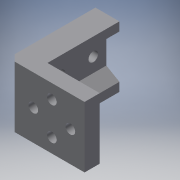
# Autodesk Inventor part: Test Mount
Saved by Autodesk Inventor 2017 (Build 210142000, 142)
## iProperties
Created: 2017-09-01
Part Number: Test Mount
Material: Generic
Document SubType Name: Modeling
Designer: Thein Lin Aung
Density: 1 g/cm^3
Appearance: Default
Author: Thein Lin Aung
Autodesk Inventor part; units mm, degrees
ref_plane "YZ Plane" through (0, 0, 0) normal (1, 0, 0) x (0, 1, 0)
ref_plane "XZ Plane" through (0, 0, 0) normal (0, 1, 0) x (-1, 0, 0)
ref_plane "XY Plane" through (0, 0, 0) normal (0, 0, 1) x (1, 0, 0)
sketch "Sketch1" plane through (0, 0, 0) normal (0, 0, 1) x (1, 0, 0)
  line L0 (35, 0) -> (0, 0)
  line L1 (0, 0) -> (0, 40)
  line L2 (0, 40) -> (5, 40)
  line L3 (5, 40) -> (5, 7)
  line L4 (5, 7) -> (35, 7)
  line L5 (35, 7) -> (35, 0)
  line L6 (-7, 0) -> (42, 0) projected
  line L7 (0, -8) -> (0, 48) projected
  dimension "d0" = 7
  dimension "d1" = 5
  dimension "d2" = 40
  dimension "d3" = 30
  constraints: 13 end point, 5 perpendicular, 1 horizontal
  measures "d0" distance of L4.end L0.start
  measures "d1" distance of L1.end L2.end
  measures "d2" distance of L0.end L1.end
  measures "d3" distance of L3.end L4.end
extrude "Extrusion1" add sketch "Sketch1" along normal mid plane 28
sketch "Sketch2" plane through (5, 7, 14) normal (0, 1, 0) x (1, 0, 0)
  circle A0 centre (15, 21.5) radius 2.2 projected
  circle A1 centre (23.5, 14) radius 2.2 projected
  circle A2 centre (15, 6.5) radius 2.2 projected
  circle A3 centre (6.5, 14) radius 2.2 projected
  point P0 (-5, 14)
extrude "Extrusion2" cut sketch "Sketch2" against normal through all
sketch "Sketch3" plane through (5, 7, 14) normal (0, 1, 0) x (1, 0, 0)
  circle A0 centre (15, 6.5) radius 2.2 projected
  circle A1 centre (15, 21.5) radius 2.2 projected
  circle A2 centre (23.5, 14) radius 2.2 projected
  circle A3 centre (6.5, 14) radius 2.2 projected
  line L0 (0, 28) -> (0, 0) projected
  line L1 (30, 0) -> (0, 0) projected
  line L2 (30, 28) -> (30, 0) projected
  line L3 (0, 28) -> (30, 28) projected
  circle A4 centre (6.5, 14) radius 3.6
  circle A5 centre (15, 21.5) radius 3.6
  circle A6 centre (23.5, 14) radius 2.2 projected
  circle A7 centre (23.5, 14) radius 3.6
  circle A8 centre (15, 6.5) radius 3.6
  point P0 (-5, 14)
  dimension "d8" = 7.2
  constraints: 4 centre point, 4 coincident, 3 equal radius
  measures "d8" diameter of A4
extrude "Extrusion3" cut sketch "Sketch3" against normal blind 4 contours A4 | A5 | A7 | A8
chamfer "Chamfer1" distance 3 angle 45 1 edges at (5, 7, 0)
sketch "Sketch4" plane through (5, 40, 14) normal (1, 0, 0) x (0, 0, -1)
  line L0 (28, 0) -> (0, 0) projected
  line L1 (14, 0) -> (14, -21)
  circle A0 centre (14, -21) radius 2.2
  circle A1 centre (14, -6) radius 2.2
  point P0 (14, -40)
  dimension "d14" = 4.4
  dimension "d15" = 15
  dimension "d16" = 6
  constraints: 2 centre point, 2 end point, 1 coincident, 1 equal radius, 1 midpoint, 1 point on line, 1 vertical
  measures "d14" diameter of A0
  measures "d15" distance of A1.centre L1.end
  measures "d16" distance from line of L0 A1.centre
extrude "Extrusion4" cut sketch "Sketch4" against normal through all
chamfer "Chamfer2" distance 3 angle 45 1 edges at (0, 0, 0)
sketch "Sketch5" plane through (0, 40, 14) normal (0, 1, 0) x (1, 0, 0)
  line L0 (5, 28) -> (5, 0) projected
  line L1 (5, 28) -> (11, 28)
  line L2 (35, 28) -> (3, 28) projected
  line L3 (11, 24) -> (5, 20.5359)
  line L4 (11, 28) -> (11, 24)
  point P0 (0, 14)
  dimension "d22" = 60
  dimension "d23" = 6
  dimension "d24" = 4
  constraints: 6 end point, 2 point on line, 1 perpendicular
  measures "d22" angle of L0 L3
  measures "d23" distance of L0.start L1.end
  measures "d24" distance of L1.end L3.start
extrude "Extrusion5" add sketch "Sketch5" against normal up to surface (33 mm away)
mirror "Mirror1" about plane through (0, 0, 0) normal (0, 0, 1) of "Extrusion5"
sketch "Sketch6" plane through (0, 40, -14) normal (-1, 0, 0) x (0, 0, 1)
  line L0 (0, 0) -> (28, 0) projected
  line L1 (8, 0) -> (20, 0)
  line L2 (20, 0) -> (20, -26)
  line L3 (20, -26) -> (8, -26)
  line L4 (8, -26) -> (8, 0)
  circle A0 centre (14, -21) radius 2.2 projected
  point P0 (14, -40)
  point P1 (14, 0)
  dimension "d27" = 12
  dimension "d28" = 5
  constraints: 8 end point, 2 midpoint, 2 parallel, 1 horizontal, 1 perpendicular, 1 point on line
  measures "d27" distance of L2.end L3.end
  measures "d28" distance from line of A0.centre L3
split_face "Split1"
body "Solid1"
